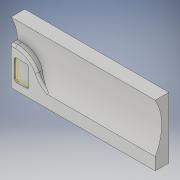
# Autodesk Inventor part: prototype #1
Saved by Autodesk Inventor 2018 (Build 220112000, 112)
## iProperties
Created: 2017-11-02
Part Number: prototype #1
Material: Generic
Document SubType Name: Modeling
Designer: 990813
Density: 1 g/cm^3
Appearance: Default
Author: 990813
Autodesk Inventor part; units mm, degrees
ref_plane "YZ Plane" through (0, 0, 0) normal (1, 0, 0) x (0, 1, 0)
ref_plane "XZ Plane" through (0, 0, 0) normal (0, 1, 0) x (-1, 0, 0)
ref_plane "XY Plane" through (0, 0, 0) normal (0, 0, 1) x (1, 0, 0)
sketch "Sketch1" plane through (0, 0, 0) normal (0, 0, 1) x (1, 0, 0)
  line L0 (0, 0) -> (200, 0)
  line L1 (200, 0) -> (200, 85)
  line L2 (200, 85) -> (0, 85)
  line L3 (0, 85) -> (0, 0)
  dimension "d0" = 200
  dimension "d1" = 85
  constraints: 8 end point, 2 parallel, 1 horizontal, 1 perpendicular
  measures "d0" distance of L2.end L1.end
  measures "d1" distance of L1.end L0.end
extrude "Extrusion1" add sketch "Sketch1" along normal blind 19
sketch "Sketch2" plane through (200, 0, 0) normal (1, 0, 0) x (0, 0, -1)
  line L0 (0, 0) -> (-19, 0)
  line L1 (0, 85) -> (-19, 85)
  line L2 (-19, 0) -> (-19, 17.145)
  line L3 (-19, 0) -> (-19, 85)
  arc A0 (-19, 17.145) -> (-19, 85) centre (-78.88828, 51.0725) ccw
  dimension "d9" = 17.145
  constraints: 2 end point, 2 point on circle, 1 centre point, 1 point on line
  measures "d9" distance of L0.end L2.end
extrude "Extrusion2" cut sketch "Sketch2" against normal through all
sketch "Sketch9" plane through (0, 0, 19) normal (0, 0, 1) x (1, 0, 0)
  line L0 (200, 17.145) -> (0, 17.145)
  line L1 (0, 17.145) -> (0, 85)
  arc A0 (39.872453, 17.145) -> (6.564985, 53.358607) centre (6.564985, 19.934531) ccw
  line L2 (0, 48.498632) -> (0, 17.145)
  line L3 (59.963777, 17.145) -> (0, 17.145)
  arc A1 (36.188235, 35.41458) -> (59.963777, 17.145) centre (63.342552, 46.147264) ccw
  line L4 (6.564985, 53.358607) -> (0, 53.358607)
  line L5 (0, 85) -> (0, 0)
  line L6 (0, 52.598177) -> (0, 53.358607)
  point P0 (39.90794, 17.607248)
  constraints: 8 end point, 6 point on circle, 5 point on line, 3 collinear, 2 centre point, 1 perpendicular, 1 tangent
extrude "Extrusion6" add sketch "Sketch9" against normal blind 12.7 contours L0 A0 A1 | L0 L1 L4 A0 A1
fillet "Fillet4" radius 3.175 2 edges at (23.8821, 48.5228, 19) (45.5518, 22.9948, 19)
sketch "Sketch12" plane through (0, 0, 19) normal (0, 0, 1) x (1, 0, 0)
  line L0 (7.239, 39.37) -> (21.209, 39.37)
  line L1 (24.384, 36.195) -> (24.384, 13.335)
  line L2 (21.209, 10.16) -> (7.239, 10.16)
  line L3 (4.064, 13.335) -> (4.064, 36.195)
  line L4 (0, 50.183607) -> (0, 0)
  line L5 (0, 0) -> (200, 0)
  arc A0 (7.239, 39.37) -> (4.064, 36.195) centre (7.239, 36.195) ccw
  arc A1 (24.384, 36.195) -> (21.209, 39.37) centre (21.209, 36.195) ccw
  arc A2 (21.209, 10.16) -> (24.384, 13.335) centre (21.209, 13.335) ccw
  arc A3 (4.064, 13.335) -> (7.239, 10.16) centre (7.239, 13.335) ccw
  point P0 (4.064, 39.37)
  point P1 (24.384, 10.16)
  point P2 (24.384, 39.37)
  point P3 (4.064, 10.16)
  dimension "d32" = 20.32
  dimension "d33" = 29.21
  dimension "d34" = 4.064
  dimension "d35" = 10.16
  dimension "d38" = 3.175
  constraints: 8 end point, 8 point on circle, 8 point on line, 8 tangent, 4 centre point, 3 equal radius, 2 parallel, 1 horizontal, 1 perpendicular
  measures "d32" distance of point (24.384, 10.16) point (4.064, 10.16)
  measures "d33" distance of point (24.384, 39.37) point (24.384, 10.16)
  measures "d34" distance between parallel lines of L4 L3
  measures "d35" distance between parallel lines of L5 L2
  measures "d38" radius of A0
extrude "Extrusion8" cut sketch "Sketch12" against normal blind 3.175
sketch "Sketch13" plane through (0, 0, 15.825) normal (0, 0, 1) x (1, 0, 0)
  line L0 (4.064, 13.335) -> (4.064, 36.195) projected
  arc A0 (4.064, 13.335) -> (7.239, 10.16) centre (7.239, 13.335) ccw projected
  line L1 (21.209, 10.16) -> (7.239, 10.16) projected
  arc A1 (21.209, 10.16) -> (24.384, 13.335) centre (21.209, 13.335) ccw projected
  line L2 (24.384, 36.195) -> (24.384, 13.335) projected
  arc A2 (24.384, 36.195) -> (21.209, 39.37) centre (21.209, 36.195) ccw projected
  line L3 (7.239, 39.37) -> (21.209, 39.37) projected
  arc A3 (7.239, 39.37) -> (4.064, 36.195) centre (7.239, 36.195) ccw projected
  point P0 (0, 0)
body "Solid1"
